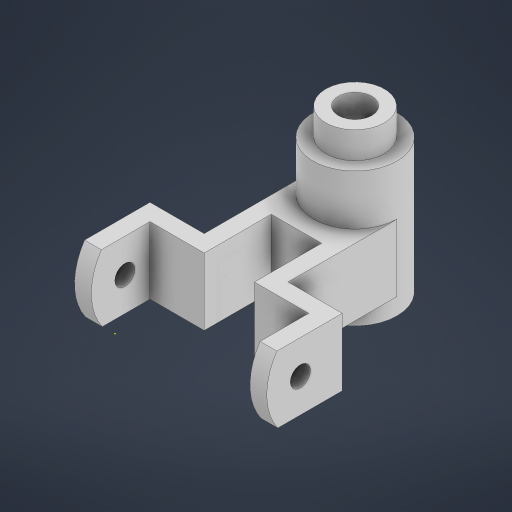
# Autodesk Inventor part: Część4
Saved by Autodesk Inventor 2023 (Build 270158000, 158)
## iProperties
Created: 2023-05-07
Part Number: Część4
Material: Ogólny
Document SubType Name: Modeling
Designer: Adam
Density: 1 g/cm^3
Appearance: Domyślna
Author: Adam
Autodesk Inventor part; units mm, degrees
ref_plane "YZ Plane" through (0, 0, 0) normal (1, 0, 0) x (0, 1, 0)
ref_plane "XZ Plane" through (0, 0, 0) normal (0, 1, 0) x (-1, 0, 0)
ref_plane "XY Plane" through (0, 0, 0) normal (0, 0, 1) x (1, 0, 0)
sketch "Szkic1" plane through (0, 0, 0) normal (0, 1, 0) x (-1, 0, 0)
  circle A0 centre (0, -143.2209) radius 25
  line L0 (25, -143.2209) -> (25, -78.2209)
  line L1 (25, -78.2209) -> (57.3466, -78.2209)
  line L2 (57.3466, -78.2209) -> (57.3466, -33.2209)
  line L3 (57.3466, -33.2209) -> (47.3466, -33.2209)
  line L4 (47.3466, -33.2209) -> (47.3466, -68.2209)
  line L5 (47.3466, -68.2209) -> (15, -68.2209)
  line L6 (15, -68.2209) -> (15, -108.2209)
  line L7 (15, -108.2209) -> (0, -108.2209)
  line L8 (0, -108.2209) -> (0, 0)
  line L9 (-25, -143.2209) -> (-25, -78.2209)
  line L10 (-25, -78.2209) -> (-57.3466, -78.2209)
  line L11 (-57.3466, -78.2209) -> (-57.3466, -33.2209)
  line L12 (-57.3466, -33.2209) -> (-47.3466, -33.2209)
  line L13 (-47.3466, -33.2209) -> (-47.3466, -68.2209)
  line L14 (-47.3466, -68.2209) -> (-15, -68.2209)
  line L15 (-15, -68.2209) -> (-15, -108.2209)
  line L16 (-15, -108.2209) -> (0, -108.2209)
  point P0 (7.5, -108.2209)
  point P1 (52.3466, -33.2209)
  dimension "d0" = 50
  dimension "d1" = 35
  dimension "d2" = 65
  dimension "d3" = 10
  dimension "d4" = 45
  dimension "d5" = 15
  dimension "d6" = 10
  dimension "d7" = 10
  constraints: 34 end point, 8 symmetric about line, 6 perpendicular, 3 vertical, 2 midpoint, 1 horizontal, 3 other
  measures "d1" vertical distance of point (7.5, -108.221) point (0, -143.221)
  measures "d2" distance from line of point (0, -143.221) L1
  measures "d3" distance between parallel lines of L5 L1
  measures "d4" distance from line of point (52.347, -33.221) L1
  measures "d5" distance of L6.end L7.end
  measures "d6" distance between parallel lines of L6 L0
  measures "d7" distance between parallel lines of L4 L2
extrude "Wyciągnięcie proste1" add sketch "Szkic1" along normal blind 40 contours A0 L9 L10 L11 L12 L13 L14 L15 L16 L7 L6 L5 L4 L3 L2 L1 L0
sketch "Szkic2" plane through (0, 40, 0) normal (0, 1, 0) x (1, 0, 0)
  point P0 (0, 0)
sketch "Szkic3" plane through (0, 40, 0) normal (0, 1, 0) x (1, 0, 0)
  circle A0 centre (0, 143.2209) radius 25
  point P0 (0, 0)
  constraints: 1 centre point
extrude "Wyciągnięcie proste2" add sketch "Szkic3" along normal blind 30 and the other way blind 50
sketch "Szkic4" plane through (0, 70, -143.2209) normal (0, 1, 0) x (1, 0, 0)
  circle A0 centre (0, 0) radius 17.5
  point P0 (0, -143.2209)
  dimension "d14" = 35
  constraints: 1 centre point
  measures "d14" diameter of A0
extrude "Wyciągnięcie proste3" add sketch "Szkic4" along normal blind 16
sketch "Szkic5" plane through (0, 86, -143.2209) normal (0, 1, 0) x (1, 0, 0)
  point P0 (0, -143.2209)
  point P1 (0, 0)
hole "Otwór1" at (0, 86, -143.2209) direction (0, -1, 0) diameter 20 end through all
sketch "Szkic6" plane through (57.3466, 0, -33.2209) normal (1, 0, 0) x (0, 0, -1)
  line L0 (0, 0) -> (0, 40) projected
  circle A0 centre (35, 20.3911) radius 35
  line L1 (0, 0) -> (0, 40) projected
  line L2 (35, 40) -> (0, 40) projected
  line L3 (6.0088, 40) -> (0, 40)
  line L4 (35, 0) -> (0, 0) projected
  line L5 (0, 40) -> (0, 0)
  line L6 (0, 0) -> (6.5535, 0)
  point P0 (-33.2209, 0)
  point P1 (0, 20.3911)
  dimension "d24" = 70
  constraints: 6 end point, 2 point on circle, 2 point on line, 1 centre point, 1 collinear, 1 tangent, 1 vertical
  measures "d24" diameter of A0
extrude "Wyciągnięcie proste4" cut sketch "Szkic6" against normal through all contours L0 A0 L4 | L0 L2 A0
sketch "Szkic7" plane through (57.3466, 0, -78.2209) normal (1, 0, 0) x (0, 0, -1)
  line L0 (-38.4465, 0) -> (0, 0) projected
  arc A0 (-38.9912, 40) -> (-38.4465, 0) centre (-10, 20.3911) ccw projected
  point P0 (-78.2209, 0)
  point P1 (-25, 20)
  dimension "d27" = 20
  dimension "d28" = 15
  measures "d27" distance from line of L0 point (-25, 20)
  measures "d28" horizontal distance of point (-25, 20) A0.centre
hole "Otwór2" at (57.3466, 20, -53.2209) direction (-1, 0, 0) diameter 12 end through all
